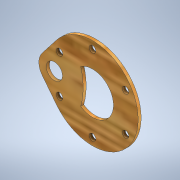
# Autodesk Inventor part: GenevaDrive
Saved by Autodesk Inventor 2020.2 (Build 242310000, 310)
## iProperties
Created: 2019-11-06
Part Number: GenevaDrive
Material: Plywood, Finish
Document SubType Name: Modeling
Designer: Paul Lefeuvre
Density: 0.552 g/cm^3
Appearance: Plywood - New
Author: Paul Lefeuvre
Autodesk Inventor part; units mm, degrees
ref_plane "YZ Plane" through (0, 0, 0) normal (1, 0, 0) x (0, 1, 0)
ref_plane "XZ Plane" through (0, 0, 0) normal (0, 1, 0) x (-1, 0, 0)
ref_plane "XY Plane" through (0, 0, 0) normal (0, 0, 1) x (1, 0, 0)
sketch "Sketch1" plane through (0, 0, 0) normal (0, 0, 1) x (1, 0, 0)
  circle A0 centre (0, 0) radius 46.3745 construction
  circle A1 centre (-38.2745, 0) radius 8.1
  circle A2 centre (0, 0) radius 38.2745 construction
  circle A3 centre (0, 38.2745) radius 3.3
  circle A4 centre (0, 0) radius 53.8745 construction
  arc A5 (-50.5731, 9.5971) -> (-50.5731, -9.5971) centre (-38.2745, 0) ccw
  line L0 (-50.5731, 9.5971) -> (-36.0873, 28.1605)
  line L1 (-50.5731, -9.5971) -> (-36.0873, -28.1605)
  line L2 (0, 0) -> (-103.0291, 0) construction
  arc A6 (-36.0873, -28.1605) -> (-36.0873, 28.1605) centre (0, 0) ccw
  circle A7 centre (-33.1467, 19.1373) radius 3.3
  circle A8 centre (-33.1467, -19.1373) radius 3.3
  circle A9 centre (0, -38.2745) radius 3.3
  circle A10 centre (33.1467, -19.1373) radius 3.3
  circle A11 centre (33.1467, 19.1372) radius 3.3
  line L3 (0, 7.3323) -> (6.35, 3.6662) construction
  line L4 (6.35, 3.6662) -> (6.35, -3.6662) construction
  line L5 (6.35, -3.6662) -> (0, -7.3323) construction
  line L6 (0, -7.3323) -> (-6.35, -3.6662) construction
  line L7 (-6.35, -3.6662) -> (-6.35, 3.6662) construction
  line L8 (-6.35, 3.6662) -> (0, 7.3323) construction
  line L9 (6.95, 4.0126) -> (0, 8.0252)
  line L10 (0, 8.0252) -> (-6.95, 4.0126)
  line L11 (-6.95, 4.0126) -> (-6.95, -4.0126)
  line L12 (-6.95, -4.0126) -> (0, -8.0252)
  line L13 (0, -8.0252) -> (6.95, -4.0126)
  line L14 (6.95, -4.0126) -> (6.95, 4.0126)
  circle A12 centre (-38.2745, 0) radius 7.5 construction
  circle A13 centre (0, 0) radius 21.6 construction
  line L15 (0, 0) -> (-246.4986, 0) construction
  line L16 (0, 0) -> (-10, 0) construction
  arc A14 (-12.528, -17.5957) -> (-12.528, 17.5957) centre (-72.5, 0) ccw construction
  arc A15 (-11.832, -17.3495) -> (-11.832, 17.3495) centre (-72.5, 0) ccw
  circle A16 centre (0, 0) radius 21
  dimension "d0" = 92.749
  dimension "d4" = 6.6
  dimension "d11" = 7.5
  dimension "d16" = 360
  dimension "d18" = 12.7
  dimension "d19" = 0.6
  dimension "d28" = 15
  dimension "d29" = 0.6
  dimension "d30" = 43.2
  dimension "d34" = 10
  dimension "d35" = 0.6
  dimension "d36" = 0.6
  dimension "d39" = 7.5
  constraints: 34 end point, 17 centre point, 16 point on circle, 6 coincident, 6 tangent, 3 point on line, 2 concentric, 2 horizontal, 32 other
  measures "d0" diameter of A0
  measures "d4" diameter of A3
  measures "d11" radial gap between concentric circles of A4 A0
  measures "d18" distance of L3.end L7.end
  measures "d19" distance between parallel lines of L3 L9
  measures "d28" diameter of A12
  measures "d29" radial gap between concentric circles of A1 A12
  measures "d30" diameter of A13
  measures "d34" distance of L15.start L16.end
  measures "d35" radial gap between concentric circles of A14 A15
  measures "d36" radial gap between concentric circles of A13 A16
  measures "d39" radial gap between concentric circles of A6 A2
extrude "Extrusion1" add sketch "Sketch1" along normal blind 3 contours L0 A6 L1 A5 | A16 A15 picked at (-13.2645, 4.6046)
body "Solid1"
